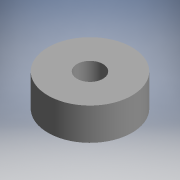
# Autodesk Inventor part: ball_bearing
Saved by Autodesk Inventor 2017 (Build 210142000, 142)
## iProperties
Part Number: ball_bearing
Material: Generic
Document SubType Name: Modeling
Designer: alex-
Appearance: Generic
bb_outer_diameter: 1,300 cm
bb_inner_diameter: 0,400 cm
bb_height: 0,500 cm
Author: alex-
Autodesk Inventor part; units mm, degrees
ref_plane "YZ Plane" through (0, 0, 0) normal (1, 0, 0) x (0, 1, 0)
ref_plane "XZ Plane" through (0, 0, 0) normal (0, 1, 0) x (-1, 0, 0)
ref_plane "XY Plane" through (0, 0, 0) normal (0, 0, 1) x (1, 0, 0)
sketch "Sketch1" plane through (0, 0, 0) normal (0, 1, 0) x (-1, 0, 0)
  circle A0 centre (0, 0) radius 6.5
  circle A1 centre (0, 0) radius 2
  dimension "bb_outer_diameter" = 13
  dimension "bb_inner_diameter" = 4
  constraints: 2 centre point, 2 coincident
  measures "bb_outer_diameter" diameter of A0
  measures "bb_inner_diameter" diameter of A1
extrude "Extrusion1" add sketch "Sketch1" along normal blind 5
body "Solid1"
